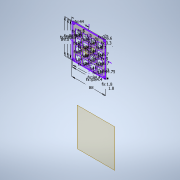
# Autodesk Inventor part: plate
Saved by Autodesk Inventor 2021 (Build 250183000, 183)
## iProperties
Created: 2020-10-02
Part Number: plate
Material: Generic
Document SubType Name: Modeling
Designer: ian66
Density: 1 g/cm^3
Appearance: Default
Author: ian66
Autodesk Inventor part; units mm, degrees
ref_plane "YZ Plane" through (0, 0, 0) normal (1, 0, 0) x (0, 1, 0)
ref_plane "XZ Plane" through (0, 0, 0) normal (0, 1, 0) x (-1, 0, 0)
ref_plane "XY Plane" through (0, 0, 0) normal (0, 0, 1) x (1, 0, 0)
ref_plane "Work Plane1" through (0, 0, 0) normal (0, 0, 1) x (1, 0, 0)
sketch "Sketch1" plane through (0, 0, 0) normal (0, 0, 1) x (1, 0, 0)
  line L0 (25.2394, 234.4042) -> (-62.7606, 234.4042)
  line L1 (-62.7606, 234.4042) -> (-62.7606, 144.9042)
  line L2 (-62.7606, 144.9042) -> (25.2394, 144.9042)
  line L3 (25.2394, 144.9042) -> (25.2394, 234.4042)
  line L4 (23.4394, 232.6042) -> (-60.9606, 232.6042)
  line L5 (-60.9606, 232.6042) -> (-60.9606, 146.7042)
  line L6 (-60.9606, 146.7042) -> (23.4394, 146.7042)
  line L7 (23.4394, 146.7042) -> (23.4394, 232.6042)
  circle A0 centre (21.9394, 231.1042) radius 3.3
  circle A1 centre (21.9394, 231.1042) radius 1.5
  line L8 (-18.7606, 249.1641) -> (-18.7606, 136.0401)
  line L9 (-67.3062, 189.6542) -> (41.0259, 189.6542)
  circle A2 centre (-59.4606, 231.1042) radius 3.3
  circle A3 centre (-59.4606, 231.1042) radius 1.5
  circle A4 centre (21.9394, 148.2042) radius 3.3
  circle A5 centre (21.9394, 148.2042) radius 1.5
  circle A6 centre (-59.4606, 148.2042) radius 3.3
  circle A7 centre (-59.4606, 148.2042) radius 1.5
  line L10 (2.7394, 221.1042) -> (16.7394, 221.1042)
  line L11 (16.7394, 221.1042) -> (16.7394, 207.1042)
  line L12 (16.7394, 207.1042) -> (2.7394, 207.1042)
  line L13 (2.7394, 207.1042) -> (2.7394, 221.1042)
  line L14 (-16.2606, 221.1042) -> (-2.2606, 221.1042)
  line L15 (-2.2606, 221.1042) -> (-2.2606, 207.1042)
  line L16 (-2.2606, 207.1042) -> (-16.2606, 207.1042)
  line L17 (-16.2606, 207.1042) -> (-16.2606, 221.1042)
  line L18 (2.7394, 202.1042) -> (16.7394, 202.1042)
  line L19 (16.7394, 202.1042) -> (16.7394, 188.1042)
  line L20 (16.7394, 188.1042) -> (2.7394, 188.1042)
  line L21 (2.7394, 188.1042) -> (2.7394, 202.1042)
  line L22 (-16.2606, 202.1042) -> (-2.2606, 202.1042)
  line L23 (-2.2606, 202.1042) -> (-2.2606, 188.1042)
  line L24 (-2.2606, 188.1042) -> (-16.2606, 188.1042)
  line L25 (-16.2606, 188.1042) -> (-16.2606, 202.1042)
  line L26 (2.7394, 183.1042) -> (16.7394, 183.1042)
  line L27 (16.7394, 183.1042) -> (16.7394, 169.1042)
  line L28 (16.7394, 169.1042) -> (2.7394, 169.1042)
  line L29 (2.7394, 169.1042) -> (2.7394, 183.1042)
  line L30 (-2.2606, 169.1042) -> (-16.2606, 169.1042)
  line L31 (-16.2606, 169.1042) -> (-16.2606, 183.1042)
  line L32 (-16.2606, 183.1042) -> (-2.2606, 183.1042)
  line L33 (-2.2606, 183.1042) -> (-2.2606, 169.1042)
  line L34 (16.7394, 150.1042) -> (2.7394, 150.1042)
  line L35 (2.7394, 150.1042) -> (2.7394, 164.1042)
  line L36 (2.7394, 164.1042) -> (16.7394, 164.1042)
  line L37 (16.7394, 164.1042) -> (16.7394, 150.1042)
  line L38 (-2.2606, 150.1042) -> (-16.2606, 150.1042)
  line L39 (-16.2606, 150.1042) -> (-16.2606, 164.1042)
  line L40 (-16.2606, 164.1042) -> (-2.2606, 164.1042)
  line L41 (-2.2606, 164.1042) -> (-2.2606, 150.1042)
  line L42 (-35.2606, 221.1042) -> (-21.2606, 221.1042)
  line L43 (-21.2606, 221.1042) -> (-21.2606, 207.1042)
  line L44 (-21.2606, 207.1042) -> (-35.2606, 207.1042)
  line L45 (-35.2606, 207.1042) -> (-35.2606, 221.1042)
  line L46 (-40.2606, 207.1042) -> (-54.2606, 207.1042)
  line L47 (-54.2606, 207.1042) -> (-54.2606, 221.1042)
  line L48 (-54.2606, 221.1042) -> (-40.2606, 221.1042)
  line L49 (-40.2606, 221.1042) -> (-40.2606, 207.1042)
  line L50 (-21.2606, 188.1042) -> (-35.2606, 188.1042)
  line L51 (-35.2606, 188.1042) -> (-35.2606, 202.1042)
  line L52 (-35.2606, 202.1042) -> (-21.2606, 202.1042)
  line L53 (-21.2606, 202.1042) -> (-21.2606, 188.1042)
  line L54 (-40.2606, 188.1042) -> (-54.2606, 188.1042)
  line L55 (-54.2606, 188.1042) -> (-54.2606, 202.1042)
  line L56 (-54.2606, 202.1042) -> (-40.2606, 202.1042)
  line L57 (-40.2606, 202.1042) -> (-40.2606, 188.1042)
  line L58 (-40.2606, 150.1042) -> (-54.2606, 150.1042)
  line L59 (-54.2606, 164.1042) -> (-40.2606, 164.1042)
  line L60 (-54.2606, 150.1042) -> (-54.2606, 164.1042)
  line L61 (-40.2606, 164.1042) -> (-40.2606, 150.1042)
  line L62 (-35.2606, 150.1042) -> (-35.2606, 164.1042)
  line L63 (-35.2606, 164.1042) -> (-21.2606, 164.1042)
  line L64 (-21.2606, 150.1042) -> (-35.2606, 150.1042)
  line L65 (-21.2606, 164.1042) -> (-21.2606, 150.1042)
  line L66 (-21.2606, 169.1042) -> (-35.2606, 169.1042)
  line L67 (-40.2606, 169.1042) -> (-54.2606, 169.1042)
  line L68 (-35.2606, 183.1042) -> (-21.2606, 183.1042)
  line L69 (-21.2606, 183.1042) -> (-21.2606, 169.1042)
  line L70 (-35.2606, 169.1042) -> (-35.2606, 183.1042)
  line L71 (-40.2606, 183.1042) -> (-40.2606, 169.1042)
  line L72 (-54.2606, 183.1042) -> (-40.2606, 183.1042)
  line L73 (-54.2606, 169.1042) -> (-54.2606, 183.1042)
  point P0 (-18.7606, 189.6542)
  point P1 (-18.7606, 234.4042)
  point P2 (-18.7606, 189.6542)
  point P3 (25.2394, 189.6542)
  dimension "d0" = 88
  dimension "d1" = 89.5
  dimension "d2" = 84.4
  dimension "d3" = 85.9
  dimension "d4" = 1.8
  dimension "d5" = 1.8
  dimension "d6" = 6.6
  dimension "d7" = 3.3
  dimension "d8" = 3.3
  dimension "d9" = 3
  dimension "d12" = 44.75
  dimension "d13" = 44
  dimension "d70" = 84.4
  dimension "d71" = 85.9
  dimension "d81" = 14
  dimension "d82" = 14
  dimension "d83" = 14
  dimension "d84" = 14
  dimension "d85" = 5
  dimension "d86" = 14
  dimension "d87" = 14
  dimension "d88" = 5
  dimension "d89" = 14
  dimension "d90" = 14
  dimension "d91" = 5
  dimension "d92" = 5
  dimension "d93" = 14
  dimension "d94" = 14
  dimension "d95" = 14
  dimension "d96" = 14
  dimension "d97" = 5
  dimension "d98" = 14
  dimension "d99" = 14
  dimension "d100" = 5
  dimension "d101" = 14
  dimension "d102" = 14
  dimension "d103" = 5
  dimension "d104" = 5
  dimension "d105" = 5
  dimension "d106" = 5
  dimension "d107" = 11.5
  dimension "d108" = 11.5
  dimension "d109" = 14
  dimension "d110" = 14
  dimension "d111" = 14
  dimension "d112" = 14
  dimension "d113" = 5
  dimension "d114" = 14
  dimension "d115" = 14
  dimension "d116" = 5
  dimension "d117" = 14
  dimension "d118" = 14
  dimension "d119" = 5
  dimension "d120" = 5
  dimension "d121" = 14
  dimension "d122" = 14
  dimension "d123" = 14
  dimension "d124" = 14
  dimension "d125" = 5
  dimension "d126" = 14
  dimension "d127" = 14
  dimension "d128" = 5
  dimension "d129" = 14
  dimension "d130" = 14
  constraints: 148 end point, 36 parallel, 19 horizontal, 18 perpendicular, 8 centre point, 6 symmetric about line, 4 coincident, 1 vertical, 6 other
  measures "d0" distance of L2.end L1.end
  measures "d1" distance of L1.end L0.end
  measures "d2" distance of L6.end L5.end
  measures "d3" distance of L5.end L4.end
  measures "d4" distance between parallel lines of L3 L7
  measures "d5" distance between parallel lines of L2 L6
  measures "d6" diameter of A0
  measures "d7" distance from line of L3 A0.centre
  measures "d8" distance from line of L0 A0.centre
  measures "d9" diameter of A1
  measures "d12" distance from line of L2 point (-18.761, 189.654)
  measures "d13" distance from line of L1 point (-18.761, 189.654)
  measures "d70" diameter of L7 L8
  measures "d71" diameter of L4 L9
  measures "d81" distance of L11.end L12.end
  measures "d82" distance of L10.end L11.end
  measures "d83" distance of L16.start L16.end
  measures "d84" distance of L14.end L16.start
  measures "d85" distance between parallel lines of L13 L15
  measures "d86" distance of L20.start L20.end
  measures "d87" distance of L18.end L20.start
  measures "d88" distance between parallel lines of L18 L12
  measures "d89" distance of L24.start L24.end
  measures "d90" distance of L22.end L24.start
  measures "d91" distance between parallel lines of L22 L16
  measures "d92" distance between parallel lines of L21 L23
  measures "d93" distance of L28.start L28.end
  measures "d94" distance of L26.end L28.start
  measures "d95" distance of L30.start L30.end
  measures "d96" distance of L33.start L30.start
  measures "d97" distance between parallel lines of L29 L33
  measures "d98" distance of L34.start L35.start
  measures "d99" distance of L36.end L34.start
  measures "d100" distance between parallel lines of L36 L28
  measures "d101" distance of L38.start L38.end
  measures "d102" distance of L40.end L38.start
  measures "d103" distance between parallel lines of L40 L30
  measures "d104" distance between parallel lines of L35 L41
  measures "d105" distance between parallel lines of L32 L24
  measures "d106" distance between parallel lines of L20 L26
  measures "d107" distance between parallel lines of L4 L10
  measures "d108" distance between parallel lines of L4 L14
  measures "d109" distance of L44.start L45.start
  measures "d110" distance of L43.start L44.start
  measures "d111" distance of L46.start L47.start
  measures "d112" distance of L49.start L46.start
  measures "d113" distance between parallel lines of L45 L49
  measures "d114" distance of L50.start L51.start
  measures "d115" distance of L53.start L50.start
  measures "d116" distance between parallel lines of L52 L44
  measures "d117" distance of L54.start L55.start
  measures "d118" distance of L57.start L54.start
  measures "d119" distance between parallel lines of L56 L46
  measures "d120" distance between parallel lines of L51 L57
  measures "d121" distance of L69.end L70.start
  measures "d122" distance of L68.end L69.end
  measures "d123" distance of L71.end L73.start
  measures "d124" distance of L72.end L71.end
  measures "d125" distance between parallel lines of L70 L71
  measures "d126" distance of L64.start L64.end
  measures "d127" distance of L63.end L64.start
  measures "d128" distance between parallel lines of L63 L66
  measures "d129" distance of L58.start L58.end
  measures "d130" distance of L59.end L58.start
extrude "Extrusion2" add sketch "Sketch1" against normal blind 1.5 contours L3 A0 L0 | A0 L4 L8 L0 | A0 L7 L4 | L3 L9 L7 A0 | A0 L7 L9 L19 L18 L21 L23 L22 L25 L8 L4 | L4 A1 L7 A0 | L4 L7 A1 | L9 L21 L18 L19 | L25 L22 L23 L9 | L10 L11 L12 L13 | L14 L15 L16 L17
hole "Hole2" at (21.9394, 231.1042, 0) direction (0, 0, -1) diameter 3 end through all countersink diameter 6 countersink angle 90
ref_plane "Work Plane4" through (-18.7606, 189.6542, -1.5) normal (1, 0, 0) x (0, 1, 0)
ref_plane "Work Plane5" through (-18.7606, 189.6542, 0) normal (0, -1, 0) x (1, 0, 0)
fillet "Fillet3" radius 3 1 edges at (25.2394, 234.4042, -0.75)
mirror "Mirror5" about plane through (-18.7606, 189.6542, 0) normal (0, -1, 0)
mirror "Mirror6" about plane through (-18.7606, 189.6542, -1.5) normal (1, 0, 0)
extrude "Extrusion3" cut sketch "Sketch1" against normal blind 1.5 contours L19 L20 L21 L9 | L9 L21 L18 L19 | L53 L50 L51 L9 | L9 L51 L52 L53 | L25 L22 L23 L9 | L9 L23 L24 L25 | L55 L56 L57 L9 | L9 L57 L54 L55 | L10 L11 L12 L13 | L14 L15 L16 L17 | L26 L27 L28 L29 | L30 L31 L32 L33 | L34 L35 L36 L37 | L38 L39 L40 L41 | L42 L43 L44 L45 | L46 L47 L48 L49 | L58 L60 L59 L61 | L62 L63 L65 L64 | L66 L70 L68 L69 | L67 L73 L72 L71
equation "\"d2\" = d0 - 2 * d4"
equation "\"d3\" = d1 - 2 * d5"
equation "\"d5\" = d4"
equation "\"d6\" = 2 * d4 + d9"
equation "\"d7\" = 0.5 * d6"
equation "\"d8\" = 0.5 * d6"
equation "\"d12\" = 0.5 * d1"
equation "\"d13\" = 0.5 * d0"
body "Solid2"
